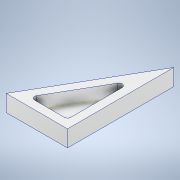
# Autodesk Inventor part: StaninaOpora.iam
Saved by Autodesk Inventor 2022 (Build 260153000, 153)
## iProperties
Created: 2023-08-15
Part Number: StaninaOpora.iam
Material: Aluminum 6061
Document SubType Name: Modeling
Designer: Kippi
Mass: 1451.62 g
Surface Area: 774.432 cm^2
Volume: 537.635 cm^3
Density: 2.7 g/cm^3
Appearance: Aluminum - Flat
Author: Kippi
Autodesk Inventor part; units mm, degrees
ref_plane "YZ Plane" through (0, 0, 0) normal (1, 0, 0) x (0, 1, 0)
ref_plane "XZ Plane" through (0, 0, 0) normal (0, 1, 0) x (-1, 0, 0)
ref_plane "XY Plane" through (0, 0, 0) normal (0, 0, 1) x (1, 0, 0)
sketch "Sketch1" plane through (0, 0, 0) normal (0, 1, 0) x (-1, 0, 0)
  line L0 (137.5, 125) -> (-10.3, 125)
  line L1 (-10.3, 125) -> (-10.3, -131)
  line L2 (-10.3, -131) -> (137.5, -131)
  line L3 (137.5, -131) -> (137.5, 125)
  line L4 (137.5, 125) -> (-10.3, -131)
  point P0 (0, 0)
  dimension "d0" = 256
  dimension "d1" = 147.8
  dimension "d7" = 30
  constraints: 10 end point, 2 parallel, 1 horizontal, 1 perpendicular
  measures "d0" distance of L0.end L1.end
  measures "d1" distance of L0.start L0.end
extrude "Extrusion1" add sketch "Sketch1" along normal blind 40 contours L4 L1 L0
sketch "Sketch2" plane through (0, 40, 0) normal (0, 1, 0) x (1, 0, 0)
  line L0 (-137.5, -125) -> (10.3, -125) construction
  line L1 (10.3, -125) -> (10.3, 131) construction
  line L2 (10.3, 131) -> (-137.5, -125) construction
  line L3 (-137.5, -125) -> (10.3, -125) construction
  line L4 (10.3, -125) -> (10.3, 131) construction
  line L5 (10.3, 131) -> (-137.5, -125) construction
  line L6 (-102.8592, -105) -> (-9.7, -105)
  line L7 (-9.7, -105) -> (-9.7, 56.3583)
  line L8 (-9.7, 56.3583) -> (-102.8592, -105)
  point P0 (0, 0)
  dimension "d4" = 20
  constraints: 6 end point, 2 other
  measures "d4" distance between parallel lines of L2 L8
extrude "Extrusion2" cut sketch "Sketch2" against normal blind 30
sketch "Sketch3" plane through (0, 10, 0) normal (0, 1, 0) x (1, 0, 0)
  line L0 (-9.7, 56.3583) -> (-9.7, -105) construction
  line L1 (-102.8592, -105) -> (-9.7, 56.3583) construction
  line L2 (-9.7, -105) -> (-102.8592, -105) construction
  point P0 (0, 0)
fillet "Fillet1" radius 8 3 edges at (-102.8592, 25, 105) (-9.7, 25, -56.3583) (-9.7, 25, 105)
body "Solid1"
